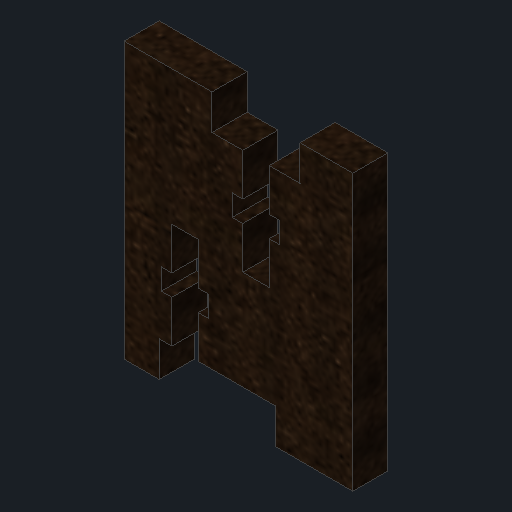
# Autodesk Inventor part: Door_LimitSwitch_Holder_Side_2
Saved by Autodesk Inventor 2024.1 (Build 281209000, 209)
## iProperties
Created: 2023-08-05
Part Number: Door_LimitSwitch_Holder_Side_2
Material: MDF Medium Density Fiberboard
Document SubType Name: Modeling
Designer: jaege
Density: 0.8 g/cm^3
Appearance: Cardboard - Corrugated
Author: jaege
Autodesk Inventor part; units mm, degrees
ref_plane "YZ Plane" through (0, 0, 0) normal (1, 0, 0) x (0, 1, 0)
ref_plane "XZ Plane" through (0, 0, 0) normal (0, 1, 0) x (-1, 0, 0)
ref_plane "XY Plane" through (0, 0, 0) normal (0, 0, 1) x (1, 0, 0)
sketch "Sketch1" plane through (0, 0, 0) normal (0, 0, 1) x (1, 0, 0)
  line L0 (-10, 4) -> (0, 4) projected
  line L1 (-10, 0) -> (-10, 4) projected
  line L2 (0, 0) -> (-10, 0) construction
  line L3 (0, 0) -> (0, 4) projected
  line L4 (10, 4) -> (12, 4) projected
  line L5 (10, 0) -> (10, 4) projected
  line L6 (12, 0) -> (10, 0) construction
  line L7 (12, 0) -> (12, 4) construction
  line L8 (12, 4) -> (12, -27.3) construction
  line L9 (12, -27.3) -> (16, -27.3) projected
  line L10 (16, 4) -> (16, -27.3) projected
  line L11 (12, 4) -> (16, 4) projected
  line L12 (6.5, 0) -> (6.5, 4) construction
  line L13 (3.5, 0) -> (3.5, 4) construction
  line L14 (6.5, 0) -> (3.5, 0) construction
  line L15 (16, -27.3) -> (-10, -27.3)
  line L16 (-10, -27.3) -> (-10, 0)
  line L17 (-10, 0) -> (16, 0) construction
  line L18 (16, 0) -> (16, -27.3)
  line L19 (0, 0) -> (10, 0)
  line L20 (3.5, 0) -> (6.5, 0)
  line L21 (6.5, 0) -> (6.5, -12)
  line L22 (6.5, -12) -> (3.5, -12)
  line L23 (3.5, -12) -> (3.5, 0)
  line L24 (2.3, -7.2) -> (7.7, -7.2)
  line L25 (7.7, -7.2) -> (7.7, -4.8)
  line L26 (7.7, -4.8) -> (2.3, -4.8)
  line L27 (2.3, -4.8) -> (2.3, -7.2)
  line L28 (-6, -27.3) -> (7.1696, -27.3)
  line L29 (7.1696, -27.3) -> (7.1696, -23.3)
  line L30 (7.1696, -23.3) -> (-6, -23.3)
  line L31 (-6, -23.3) -> (-6, -27.3)
  line L32 (-4.56, -11.3) -> (-1.56, -11.3)
  line L33 (-1.56, -11.3) -> (-1.56, -23.3)
  line L34 (-1.56, -23.3) -> (-4.56, -23.3)
  line L35 (-4.56, -23.3) -> (-4.56, -11.3)
  line L36 (-5.76, -18.5) -> (-0.36, -18.5)
  line L37 (-0.36, -18.5) -> (-0.36, -16.1)
  line L38 (-0.36, -16.1) -> (-5.76, -16.1)
  line L39 (-5.76, -16.1) -> (-5.76, -18.5)
  point P0 (2.3, -6)
  point P1 (3.5, -6)
  point P2 (5, -7.2)
  point P3 (5, -12)
  point P4 (-5.76, -17.3)
  point P5 (-4.56, -17.3)
  point P6 (-3.06, -18.5)
  point P7 (-3.06, -23.3)
  point P8 (-4.56, -18.5)
  point P9 (-4.56, -16.1)
  point P10 (-1.56, -16.1)
  point P11 (-1.56, -18.5)
  point P12 (6.5, -4.8)
  point P13 (6.5, -7.2)
  point P14 (3.5, -7.2)
  point P15 (3.5, -4.8)
  dimension "d0" = 3
  dimension "d1" = 12
  dimension "d2" = 2.4
  dimension "d3" = 5.4
  dimension "d4" = 4
  dimension "d5" = 3
  dimension "d6" = 12
  dimension "d7" = 2.4
  dimension "d8" = 5.4
  dimension "d9" = 1.44
  dimension "d10" = 4
  constraints: 54 end point, 12 parallel, 8 midpoint, 6 horizontal, 6 perpendicular, 3 horizontal alignment, 2 vertical, 2 vertical alignment, 1 collinear, 1 point on line, 4 other
  measures "d0" distance of L21.end L22.end
  measures "d1" distance of L20.end L21.end
  measures "d2" distance of L26.end L24.start
  measures "d3" distance of L24.start L24.end
  measures "d4" distance between parallel lines of L31 L16
  measures "d5" distance of L33.end L35.start
  measures "d6" distance of L33.start L33.end
  measures "d7" distance of L39.start L39.end
  measures "d8" distance of L39.end L37.start
  measures "d9" distance between parallel lines of L31 L35
  measures "d10" distance of L28.end L29.end
extrude "Extrusion1" add sketch "Sketch1" along normal blind 4 contours L0 L3 L19 L23 L26 L27 L24 L22 L21 L25 L5 L4 L11 L10 L9 L15 L29 L30 L33 L36 L37 L38 L32 L35 L39 L31 L16 L1
body "Solid1"
